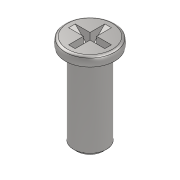
# Autodesk Inventor part: 10_047_LOW_HEAD_SCREW_M2X5_R1
Saved by Autodesk Inventor 2021.2 (Build 252289000, 289)
## iProperties
Part Number: 10_047_LOW_HEAD_SCREW_M2X5_R1
Material: ステンレス鋼
Document SubType Name: Modeling
Designer: y6tada
Density: 8 g/cm^3
Appearance: ステンレス - ブラシ仕上げ
Author: y6tada
Autodesk Inventor part; units mm, degrees
ref_plane "YZ Plane" through (0, 0, 0) normal (1, 0, 0) x (0, 1, 0)
ref_plane "XZ Plane" through (0, 0, 0) normal (0, 1, 0) x (-1, 0, 0)
ref_plane "XY Plane" through (0, 0, 0) normal (0, 0, 1) x (1, 0, 0)
sketch "スケッチ1" plane through (0, 0, 0) normal (0, 0, 1) x (1, 0, 0)
  line L0 (0, 0) -> (0, 5.2414) construction
  line L1 (1.45, 0.65) -> (1.45, 0) construction
  line L2 (1.45, 0) -> (1, 0)
  line L3 (1, 0) -> (1, -5)
  line L4 (1, -5) -> (0, -5)
  line L5 (0, -5) -> (0, 0)
  line L6 (0, 0) -> (0, 0.65)
  line L7 (1.45, 0.65) -> (0, 0.65)
  arc A0 (1.45, 0) -> (1.45, 0.65) centre (0.9719, 0.325) ccw
  line L8 (1.55, 1.278) -> (1.55, -0.8189) construction
  dimension "d0" = 2
  dimension "d1" = 5
  dimension "d2" = 3.1
  dimension "d3" = 0.1
  dimension "d4" = 0.65
  constraints: 18 end point, 4 perpendicular, 2 point on circle, 2 point on line, 2 vertical, 1 centre point, 1 horizontal, 1 tangent
  measures "d0" diameter of L3 L0
  measures "d1" distance of L2.end L3.end
  measures "d2" diameter of L8 L0
  measures "d3" distance between parallel lines of L8 L1
  measures "d4" distance between parallel lines of L7 L2
revolve "回転1" add sketch "スケッチ1" angle 360 about axis through (0, 0, 0) along (0, 1, 0)
sketch "スケッチ2" plane through (0, 0, 0) normal (0, 0, 1) x (1, 0, 0)
  line L0 (-1.45, 0.65) -> (1.45, 0.65) construction
  line L1 (1.1, 0.65) -> (0.2, -0.25)
  line L2 (0.2, -0.25) -> (0, -0.25)
  line L3 (0, -0.25) -> (0, 0.65)
  line L4 (0, 0) -> (0, -0.4614) construction
  line L5 (0, 0.65) -> (1.1, 0.65)
  dimension "d6" = 45
  dimension "d8" = 0.2
  dimension "d15" = 2.2
  constraints: 10 end point, 2 point on line, 1 collinear, 1 horizontal, 1 midpoint, 1 perpendicular, 1 vertical
  measures "d6" angle of L1 L0
  measures "d8" distance of L1.end L2.end
  measures "d15" diameter of L1.start L4
extrude "押し出し1" cut sketch "スケッチ2" along normal mid plane 0.4
pattern_circular "円形状パターン1" count 4 over 360 about axis through (0, -10, 0) along (0, 1, 0) of "押し出し1"
chamfer "面取り1" distance 0.2 angle 45 1 edges at (-1, -5, 0)
fillet "フィレット2" radius 0.15 2 edges at (-1.45, 0.65, 0) (-1.45, 0, 0)
